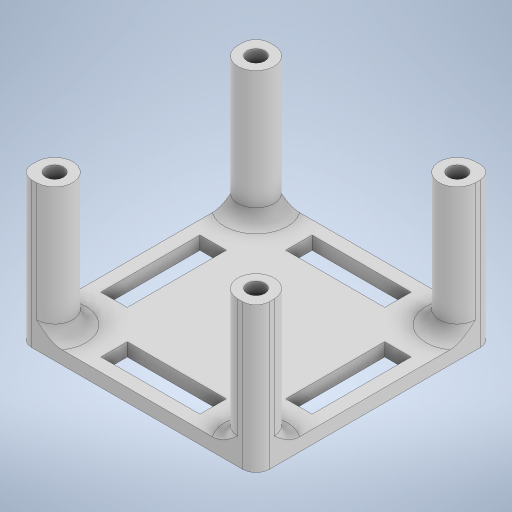
# Autodesk Inventor part: v3_gps_stand
Saved by Autodesk Inventor 2024 (Build 280153000, 153)
## iProperties
Created: 2025-07-04
Part Number: v3_gps_stand
Material: Generic
Document SubType Name: Modeling
Designer: Bruno
Density: 1 g/cm^3
Appearance: Default
Author: Bruno
Autodesk Inventor part; units mm, degrees
ref_plane "YZ Plane" through (0, 0, 0) normal (1, 0, 0) x (0, 1, 0)
ref_plane "XZ Plane" through (0, 0, 0) normal (0, 1, 0) x (-1, 0, 0)
ref_plane "XY Plane" through (0, 0, 0) normal (0, 0, 1) x (1, 0, 0)
sketch "Sketch1" plane through (0, 0, 0) normal (0, 1, 0) x (-1, 0, 0)
  line L0 (16, -18) -> (-16, -18)
  line L1 (-18, -16) -> (-18, 16)
  line L2 (-16, 18) -> (16, 18)
  line L3 (18, 16) -> (18, -16)
  line L4 (18, -18) -> (-18, 18)
  circle A0 centre (-15.25, -15.25) radius 1.35
  line L5 (0, -18) -> (0, 18)
  line L6 (18, 0) -> (-18, 0)
  circle A1 centre (-15.25, 15.25) radius 1.35
  circle A2 centre (15.25, -15.25) radius 1.35
  circle A3 centre (15.25, 15.25) radius 1.35
  arc A4 (16, -18) -> (18, -16) centre (16, -16) ccw
  arc A5 (-18, -16) -> (-16, -18) centre (-16, -16) ccw
  arc A6 (-16, 18) -> (-18, 16) centre (-16, 16) ccw
  arc A7 (18, 16) -> (16, 18) centre (16, 16) ccw
  point P0 (0, 0)
  point P1 (-18, -18)
  point P2 (18, 18)
  point P3 (0, 0)
  dimension "d0" = 36
  dimension "d1" = 36
  dimension "d4" = 2.7
  dimension "d5" = 30.5
  dimension "d6" = 30.5
  dimension "d7" = 2
  constraints: 14 end point, 8 centre point, 8 point on circle, 8 point on line, 8 tangent, 5 midpoint, 3 equal radius, 3 symmetric about line, 2 parallel, 1 coincident, 1 horizontal, 1 perpendicular, 3 other
  measures "d0" distance of L4.start point (-18, -18)
  measures "d1" distance of point (-18, -18) L4.end
  measures "d4" diameter of A0
  measures "d5" diameter of A0.centre L6
  measures "d6" diameter of A0.centre L5
  measures "d7" radius of A4
extrude "Extrusion1" add sketch "Sketch1" along normal blind 2 contours L0 L5 L4 A2 A4 | L0 A5 L1 L6 L5 | L4 A2 L6 L3 A4 | L6 L1 A6 L4 A1 | L4 A1 A6 L2 L5 | L5 L2 A7 L3 L6
sketch "Sketch2" plane through (0, 2, 0) normal (0, 1, 0) x (1, 0, 0)
  circle A0 centre (-15.25, 15.25) radius 1.35 projected
  circle A1 centre (15.25, 15.25) radius 1.35 projected
  circle A2 centre (-15.25, -15.25) radius 1.35 projected
  circle A3 centre (15.25, -15.25) radius 1.35 projected
  circle A4 centre (-15.25, 15.25) radius 2.75
  line L0 (16, 18) -> (-16, 18) projected
  line L1 (0, 18) -> (0, -18)
  line L2 (-16, -18) -> (16, -18) projected
  line L3 (18, -16) -> (18, 16) projected
  line L4 (18, 0) -> (-18, 0)
  line L5 (-18, 16) -> (-18, -16) projected
  arc A5 (-16, 18) -> (-18, 16) centre (-16, 16) ccw projected
  line L6 (-16, -18) -> (16, -18) projected
  arc A6 (16, -18) -> (18, -16) centre (16, -16) ccw projected
  line L7 (18, -16) -> (18, 16) projected
  arc A7 (18, 16) -> (16, 18) centre (16, 16) ccw projected
  line L8 (16, 18) -> (-16, 18) projected
  arc A8 (-16, 18) -> (-18, 16) centre (-16, 16) ccw projected
  line L9 (-18, 16) -> (-18, -16) projected
  arc A9 (-18, -16) -> (-16, -18) centre (-16, -16) ccw projected
  circle A10 centre (15.25, 15.25) radius 1.35 projected
  circle A11 centre (-15.25, 15.25) radius 1.35 projected
  circle A12 centre (-15.25, -15.25) radius 1.35 projected
  circle A13 centre (15.25, -15.25) radius 1.35 projected
  circle A14 centre (15.25, 15.25) radius 2.75
  circle A15 centre (-15.25, -15.25) radius 2.75
  circle A16 centre (15.25, -15.25) radius 2.75
  point P0 (0, 0)
  point P1 (18, -15.25)
  point P2 (15.25, -18)
  point P3 (-15.25, -18)
  point P4 (-18, -15.25)
  point P5 (-18, -16)
  point P6 (15.25, 18)
  point P7 (18, 15.25)
  point P8 (-15.25, 18)
  point P9 (-18, 15.25)
  constraints: 4 centre point, 4 end point, 4 midpoint, 3 symmetric about line, 1 coincident, 1 tangent, 3 other
extrude "Extrusion2" add sketch "Sketch2" along normal blind 20 contours A4 | A4 L5 A5 L0 | L0 A7 L3 A14 | A14 | A15 L2 A9 L5 | A15 | A16 L3 A6 L2 | A16
fillet "Fillet1" radius 2 4 edges at (-13.3055, 2, 13.3055) (13.3055, 2, 13.3055) (13.3055, 2, -13.3055) (-13.3055, 2, -13.3055)
sketch "Sketch3" plane through (0, 0, 0) normal (0, -1, 0) x (1, 0, 0)
  line L0 (-7.5, 16) -> (7.5, 16)
  line L1 (7.5, 16) -> (7.5, 12)
  line L2 (7.5, 12) -> (-7.5, 12)
  line L3 (-7.5, 12) -> (-7.5, 16)
  line L4 (-7.5, 12) -> (7.5, 16)
  line L5 (-16, 18) -> (16, 18) projected
  line L6 (0, 18) -> (0, -18)
  line L7 (11.377, -18) -> (-11.377, -18) projected
  line L8 (16, 7.5) -> (16, -7.5)
  line L9 (12, 7.5) -> (16, 7.5)
  line L10 (12, -7.5) -> (12, 7.5)
  line L11 (16, -7.5) -> (12, -7.5)
  line L12 (7.5, -16) -> (-7.5, -16)
  line L13 (7.5, -12) -> (7.5, -16)
  line L14 (-7.5, -12) -> (7.5, -12)
  line L15 (-7.5, -16) -> (-7.5, -12)
  line L16 (-16, -7.5) -> (-16, 7.5)
  line L17 (-12, -7.5) -> (-16, -7.5)
  line L18 (-12, 7.5) -> (-12, -7.5)
  line L19 (-16, 7.5) -> (-12, 7.5)
  point P0 (0, 0)
  point P1 (0, 14)
  point P2 (0, -12)
  point P3 (0, -16)
  dimension "d11" = 4
  dimension "d12" = 4
  dimension "d13" = 15
  dimension "d16" = 360
  constraints: 36 end point, 3 midpoint, 2 parallel, 1 horizontal, 1 perpendicular, 1 point on line, 33 other
  measures "d11" diameter of L0 L5
  measures "d12" distance of L0.end L1.end
  measures "d13" distance of L0.start L0.end
extrude "Extrusion3" cut sketch "Sketch3" against normal through all
body "Solid1"
